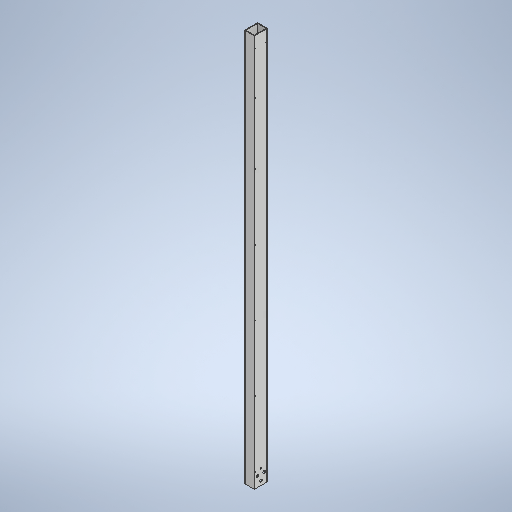
# Autodesk Inventor part: profil_stalowy_40_30_120
Saved by Autodesk Inventor 2025.2 (Build 292293000, 293)
## iProperties
Created: 2025-03-18
Part Number: profil_stalowy_40_30_120
Material: Ogólny
Document SubType Name: Modeling
Designer: tadek
Density: 1 g/cm^3
Appearance: Domyślna
Author: tadek
Autodesk Inventor part; units mm, degrees
ref_plane "YZ Plane" through (0, 0, 0) normal (1, 0, 0) x (0, 1, 0)
ref_plane "XZ Plane" through (0, 0, 0) normal (0, 1, 0) x (-1, 0, 0)
ref_plane "XY Plane" through (0, 0, 0) normal (0, 0, 1) x (1, 0, 0)
sketch "Szkic2" plane through (0, 0, 0) normal (0, 1, 0) x (-1, 0, 0)
  line L0 (0, 0) -> (-15, 0) construction
  line L1 (-15, 0) -> (-15, 20)
  line L2 (-15, 20) -> (0, 20)
  line L3 (-15, 0) -> (-15, -20)
  line L4 (-15, -20) -> (0, -20)
  line L5 (0, -20) -> (0, 20) construction
  line L6 (15, 0) -> (15, 20)
  line L7 (15, 20) -> (0, 20)
  line L8 (15, -20) -> (0, -20)
  line L9 (15, 0) -> (15, -20)
  line L10 (15, 0) -> (13, 0) construction
  line L11 (0, 20) -> (0, 18) construction
  line L12 (0, 18) -> (13, 18)
  line L13 (13, 18) -> (13, 0)
  line L14 (0, 18) -> (-13, 18)
  line L15 (-13, 18) -> (-13, 0)
  line L16 (0, -18) -> (13, -18)
  line L17 (13, -18) -> (13, 0)
  line L18 (-13, -18) -> (-13, 0)
  line L19 (0, -18) -> (-13, -18)
  point P0 (-7.5, -20)
  point P1 (15, -10)
  dimension "d18" = 40
  dimension "d19" = 30
  dimension "d22" = 2
  dimension "d23" = 2
  constraints: 40 end point, 10 symmetric about line, 3 midpoint, 3 perpendicular, 2 horizontal, 1 parallel, 1 point on line, 1 vertical
  measures "d18" distance from line of point (-7.5, -20) L2
  measures "d19" distance from line of L3 point (15, -10)
  measures "d22" distance of L9.start L10.end
  measures "d23" distance of L2.end L11.end
extrude "Wyciągnięcie proste4" add sketch "Szkic2" along normal blind 1200
sketch "Szkic3" plane through (15, 0, -20) normal (0, 0, -1) x (-1, 0, 0)
  line L0 (0, 1200) -> (0, 1180) construction
  line L1 (0, 0) -> (0, 1200) projected
  line L2 (0, 1180) -> (12, 1180) construction
  line L3 (12, 1180) -> (12, 0)
  line L4 (0, 0) -> (0, 1200) projected
  line L5 (0, 0) -> (0, 20)
  line L6 (0, 20) -> (12, 20)
  point P0 (15, 0)
  dimension "d26" = 20
  dimension "d27" = 12
  dimension "d76" = 1180
  dimension "d77" = 20
  constraints: 10 end point, 3 point on line, 2 perpendicular, 1 parallel
  measures "d26" distance of L0.start L0.end
  measures "d27" distance of L0.end L2.end
  measures "d76" distance of L2.end L3.end
  measures "d77" distance of L1.start L5.end
hole "Otwór1" at (3, 1180, -20) at (3, 20, -20) direction (0, 0, 1) diameter 8 depth 10 tip angle 118
sketch "Szkic4" plane through (15, 0, 20) normal (1, 0, 0) x (0, 0, -1)
  line L0 (40, 0) -> (0, 0) projected
  line L1 (0, 0) -> (10, 0)
  line L2 (40, 0) -> (30, 0)
  line L3 (0, 0) -> (0, 31)
  line L4 (0, 0) -> (0, 1200) projected
  line L5 (0, 31) -> (10, 31)
  line L6 (40, 0) -> (40, 1200) projected
  line L7 (40, 0) -> (40, 31)
  line L8 (30, 31) -> (40, 31)
  line L9 (40, 31) -> (40, 0)
  line L10 (0, 0) -> (0, 40)
  line L11 (20, 0) -> (20, 13)
  dimension "d35" = 10
  dimension "d36" = 10
  dimension "d37" = 31
  dimension "d38" = 20
  dimension "d39" = 31
  dimension "d40" = 10
  dimension "d41" = 40
  dimension "d42" = 13
  constraints: 18 end point, 5 point on line, 2 perpendicular, 1 collinear, 1 vertical
  measures "d35" distance of L0.end L1.end
  measures "d36" distance of L0.start L2.end
  measures "d37" distance of L0.end L3.end
  measures "d38" distance of L5.end L8.start
  measures "d39" distance between parallel lines of L0 L8
  measures "d40" distance from line of L8.start L6
  measures "d41" distance of L0.end L10.end
  measures "d42" distance of L11.start L11.end
hole "Otwór2" at (15, 31, 10) at (15, 31, -10) at (15, 13, 0) direction (-1, 0, 0) diameter 8 depth 8.25 tip angle 118
sketch "Szkic5" plane through (15, 0, 20) normal (1, 0, 0) x (0, 0, -1)
  line L0 (40, 0) -> (0, 0) projected
  line L1 (0, 0) -> (0, 45)
  line L2 (0, 0) -> (0, 1200) projected
  line L3 (0, 45) -> (20, 45)
  point P0 (20, 0)
  dimension "d50" = 45
  constraints: 4 end point, 1 perpendicular, 1 point on line
  measures "d50" distance of L0.end L1.end
hole "Otwór3" at (15, 45, 0) direction (-1, 0, 0) diameter 5 depth 8 tip angle 118
sketch "Szkic6" plane through (15, 0, 20) normal (1, 0, 0) x (0, 0, -1)
  line L0 (0, 0) -> (0, 1200) projected
  circle A0 centre (20, 45) radius 2.5 projected
  line L1 (0, 45) -> (3, 45)
  line L2 (3, 45) -> (3, 245)
  line L3 (3, 245) -> (3, 445)
  line L4 (3, 445) -> (3, 645)
  line L5 (3, 645) -> (3, 845)
  line L6 (3, 845) -> (3, 1035)
  line L7 (40, 1200) -> (0, 1200) projected
  line L8 (20, 0) -> (20, 1200)
  line L9 (0, 1165) -> (4, 1165)
  point P0 (2, 1200)
  point P1 (37, 45)
  point P2 (37, 245)
  point P3 (37, 445)
  point P4 (37, 645)
  point P5 (37, 845)
  point P6 (37, 1035)
  point P7 (36, 1165)
  dimension "d58" = 20
  dimension "d59" = 3
  dimension "d60" = 200
  dimension "d61" = 200
  dimension "d62" = 200
  dimension "d63" = 200
  dimension "d64" = 190
  dimension "d73" = 35
  dimension "d75" = 4
  constraints: 16 end point, 7 point on line, 7 symmetric about line, 1 horizontal, 1 midpoint, 1 perpendicular, 1 vertical
  measures "d58" distance from line of L0 A0.centre
  measures "d59" distance of L1.start L1.end
  measures "d60" distance of L1.end L2.end
  measures "d61" distance of L2.end L3.end
  measures "d62" distance of L3.end L4.end
  measures "d63" distance of L4.end L5.end
  measures "d64" distance of L5.end L6.end
  measures "d73" distance from line of L7 L9.end
  measures "d75" distance of L9.start L9.end
hole "Otwór4" at (15, 45, 17) at (15, 245, 17) at (15, 445, 17) at (15, 645, 17) at (15, 845, 17) at (15, 1035, 17) at (15, 1165, 16) at (15, 1165, -16) at (15, 1035, -17) at (15, 845, -17) at (15, 645, -17) at (15, 445, -17) at (15, 245, -17) at (15, 45, -17) direction (-1, 0, 0) diameter 2.5 depth 8 tip angle 118
